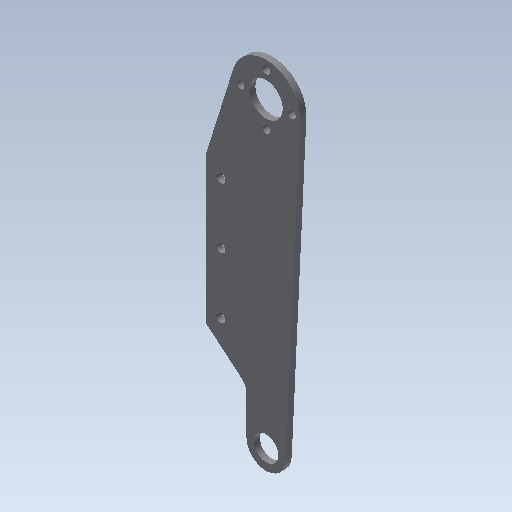
# Autodesk Inventor part: リンク_ふくらはぎ_メインフレーム_1_1
Saved by Autodesk Inventor 2020.4 (Build 244396000, 396)
## iProperties
Created: 2016-04-29
Part Number: リンク_ふくらはぎ_メインフレーム_1_1
Material: GFRP
Document SubType Name: Modeling
Designer: hiroaki
Density: 1.75 g/cm^3
Appearance: 滑らか - 淡い灰色
Mass: 9.06341 g
Surface Area: 59.5321 cm^2
Volume: 5.17909 cm^3
d0: 1.000 ul
d1: 13.000 mm
d2: 11.100 mm
d7: 3.100 mm
d8: 5.000 mm
d9: 15.000 mm
d10: 4.000 mm
d11: 40.000 mm
d12: 30.000 mm
d13: 2.000 mm
d14: 0.00 deg
d15: 2.700 mm
d16: 45.00 deg
d17: 2.700 mm
d18: 4.000 ul
d22: 1.500 mm
d23: 130.00 deg
d24: 4.000 mm
Author: hiroaki
Autodesk Inventor part; units mm, degrees
ref_plane "YZ Plane" through (0, 0, 0) normal (1, 0, 0) x (0, 1, 0)
ref_plane "XZ Plane" through (0, 0, 0) normal (0, 1, 0) x (-1, 0, 0)
ref_plane "XY Plane" through (0, 0, 0) normal (0, 0, 1) x (1, 0, 0)
derived "下半身全体像_1_1.ipt"
sketch "スケッチ1" plane through (0, 0, 0) normal (0, 0, 1) x (1, 0, 0)
  circle A0 centre (0, 0) radius 10.5 construction
  line L0 (0, 0) -> (-12, 0) construction
  arc A1 (0, 16) -> (-12, 10.583) centre (0, 0) ccw construction
  arc A2 (-12, -10.583) -> (0, -16) centre (0, 0) ccw construction
  line L1 (0, 16) -> (39.5, 16) construction
  line L2 (39.5, 16) -> (39.5, -16) construction
  line L3 (39.5, -16) -> (0, -16) construction
  circle A3 centre (1, 13.5) radius 1.35
  circle A4 centre (1, -13.5) radius 1.35 construction
  circle A5 centre (28, 13.5) radius 1.35
  circle A6 centre (28, -13.5) radius 1.35
  line L4 (1, 13.5) -> (1, -13.5) construction
  line L5 (1, -13.5) -> (28, -13.5) construction
  line L6 (1, 13.5) -> (28, 13.5) construction
  line L7 (28, 13.5) -> (28, -13.5) construction
  line L8 (0, 0) -> (1, 0) construction
  line L9 (32, 120) -> (32, 20) construction
  line L10 (0, 0) -> (0, 0) construction
  circle A7 centre (32, 120) radius 4.05
  line L11 (0, 140) -> (0, 40) construction
  circle A8 centre (0, 40) radius 4.05
  line L12 (0, 0) -> (0, -100) construction
  line L13 (32, 20) -> (32, -80) construction
  line L14 (0, 0) -> (0, 40) construction
  circle A9 centre (32, 20) radius 6.5 construction
  line L15 (32, 23.5218) -> (35.05, 21.7609) construction
  line L16 (35.05, 21.7609) -> (35.05, 18.2391) construction
  line L17 (35.05, 18.2391) -> (32, 16.4782) construction
  line L18 (32, 16.4782) -> (28.95, 18.2391) construction
  line L19 (28.95, 18.2391) -> (28.95, 21.7609) construction
  line L20 (28.95, 21.7609) -> (32, 23.5218) construction
  line L21 (21.5, 152) -> (61, 152) construction
  line L22 (61, 152) -> (61, 100.5) construction
  line L23 (61, 100.5) -> (21.5, 100.5) construction
  line L24 (21.5, 100.5) -> (21.5, 152) construction
  line L25 (21.5, 140) -> (61, 140) construction
  line L26 (16, 150.5) -> (66.5, 150.5) construction
  line L27 (66.5, 150.5) -> (66.5, 129.5) construction
  line L28 (66.5, 129.5) -> (16, 129.5) construction
  line L29 (16, 129.5) -> (16, 150.5) construction
  circle A10 centre (0, 140) radius 10.5 construction
  line L30 (-13.5, 139) -> (13.5, 139) construction
  line L31 (13.5, 139) -> (13.5, 112) construction
  line L32 (13.5, 112) -> (-13.5, 112) construction
  line L33 (-13.5, 112) -> (-13.5, 139) construction
  circle A11 centre (-13.5, 139) radius 1.35
  circle A12 centre (13.5, 139) radius 1.35
  circle A13 centre (-13.5, 112) radius 1.35
  circle A14 centre (13.5, 112) radius 1.35
  line L34 (-12, 10.583) -> (-12, -10.583) construction
  circle A15 centre (0, -100) radius 4.05
  circle A16 centre (32, -80) radius 4.05
  circle A17 centre (0, -100) radius 10.5 construction
  line L35 (32, -80) -> (0, -100) construction
  line L36 (45, -60.5) -> (77.5, -60.5) construction
  line L37 (77.5, -60.5) -> (77.5, -112) construction
  line L38 (77.5, -112) -> (45, -112) construction
  line L39 (45, -112) -> (45, -60.5) construction
  line L40 (45, -100) -> (77.5, -100) construction
  line L41 (39.5, -89.5) -> (83, -89.5) construction
  line L42 (83, -89.5) -> (83, -110.5) construction
  line L43 (83, -110.5) -> (39.5, -110.5) construction
  line L44 (39.5, -110.5) -> (39.5, -89.5) construction
  line L45 (1, -86.5) -> (28, -86.5) construction
  line L46 (28, -86.5) -> (28, -113.5) construction
  line L47 (28, -113.5) -> (1, -113.5) construction
  line L48 (1, -113.5) -> (1, -86.5) construction
  circle A18 centre (1, -86.5) radius 1.35
  circle A19 centre (1, -113.5) radius 1.35
  circle A20 centre (28, -113.5) radius 1.35
  circle A21 centre (28, -86.5) radius 1.35
  circle A22 centre (32, 20) radius 4.05
  circle A23 centre (32, 20) radius 4.05
  line L49 (10.583, 152) -> (-10.583, 152) construction
  line L50 (16, 140) -> (16, 100.5) construction
  line L51 (16, 100.5) -> (-16, 100.5) construction
  line L52 (-16, 100.5) -> (-16, 140) construction
  arc A24 (16, 140) -> (10.583, 152) centre (0, 140) ccw construction
  arc A25 (-10.583, 152) -> (-16, 140) centre (0, 140) ccw construction
  line L53 (-12, -89.417) -> (-12, -110.583) construction
  line L54 (0, -84) -> (39.5, -84) construction
  line L55 (39.5, -84) -> (39.5, -116) construction
  line L56 (39.5, -116) -> (0, -116) construction
  arc A26 (0, -84) -> (-12, -89.417) centre (0, -100) ccw construction
  arc A27 (-12, -110.583) -> (0, -116) centre (0, -100) ccw construction
  circle A28 centre (-8.5, 0) radius 1.35 construction
  circle A29 centre (0, 0) radius 8.5 construction
  line L57 (35.05, 121.7609) -> (35.05, 118.2391) construction
  line L58 (35.05, 118.2391) -> (32, 116.4782) construction
  line L59 (32, 116.4782) -> (28.95, 118.2391) construction
  line L60 (28.95, 118.2391) -> (28.95, 121.7609) construction
  line L61 (28.95, 121.7609) -> (32, 123.5218) construction
  line L62 (32, 123.5218) -> (35.05, 121.7609) construction
  circle A30 centre (0, -100) radius 6.5 construction
  circle A31 centre (0, 0) radius 5.55
  line L63 (6.4924, -100.3153) -> (11.3366, -0.5505)
  arc A32 (11.3366, -0.5505) -> (-10.8351, 3.3799) centre (0, 0) ccw
  line L64 (-10.8351, 3.3799) -> (-20, -26)
  line L65 (-20, -26) -> (-20, -74)
  arc A33 (-6.5, -100) -> (6.4924, -100.3153) centre (0, -100) ccw
  line L66 (-6.5, -100) -> (-6.5, -85.3278)
  circle A34 centre (-15, -30) radius 1.55
  line L67 (-15, -30) -> (-15, -70) construction
  circle A35 centre (-15, -70) radius 1.55
  circle A36 centre (-15, -50) radius 1.55
  line L68 (-15, -70) -> (-20, -70) construction
  line L69 (-15, -50) -> (-20, -50) construction
  line L70 (0, 152) -> (0, 140) construction
  line L71 (0, 140) -> (0, 139) construction
  circle A37 centre (-8.5, 0) radius 1.35
  line L72 (0, 0) -> (-8.5, 0) construction
  line L73 (0, 0) -> (-6.0104, 6.0104) construction
  circle A38 centre (-6.0104, 6.0104) radius 1.35
  circle A39 centre (0, -8.5) radius 1.35
  circle A40 centre (-6.0104, -6.0104) radius 1.35
  circle A41 centre (8.5, 0) radius 1.35
  circle A42 centre (6.0104, -6.0104) radius 1.35
  circle A43 centre (0, 8.5) radius 1.35
  circle A44 centre (6.0104, 6.0104) radius 1.35
  circle A45 centre (0, 0) radius 9.85 construction
  circle A46 centre (0, 0) radius 11.35 construction
  line L74 (-20, -74) -> (-6.5, -85.3278)
  line L75 (0, 0) -> (0, 8.5) construction
  point P0 (66.5, 140)
  point P1 (39.5, 0)
  point P2 (83, -100)
  point P3 (1, -100)
  point P4 (-12, -100)
  point P5 (39.5, -100)
  dimension "d1" = 13
  dimension "d2" = 11.1
  dimension "d7" = 3.1
  dimension "d8" = 5
  dimension "d9" = 15
  dimension "d10" = 4
  dimension "d11" = 40
  dimension "d12" = 30
  dimension "d15" = 2.7
  dimension "d16" = 45
  dimension "d17" = 2.7
  dimension "d20" = 360
  dimension "d22" = 1.5
  dimension "d23" = 130
  measures "d1" diameter of A30
  measures "d2" diameter of A31
  measures "d7" diameter of A34
  measures "d8" distance between parallel lines of L65 L67
  measures "d9" distance between parallel lines of L12 L67
  measures "d10" distance from line of L65.end L68
  measures "d11" distance of L67.start L67.end
  measures "d12" distance from line of A30.centre L68
  measures "d15" diameter of A37
  measures "d16" angle of L72 L73
  measures "d17" diameter of A38
  measures "d22" radial gap between concentric circles of A46 A45
  measures "d23" angle of L65 L74
extrude "押し出し1" add sketch "スケッチ1" along normal blind 2 contours A18 | A33 L66 L74 L65 L64 A32 L63 | A38 | A40 | A42 | A44
fillet "フィレット1" radius 4 1 edges at (-6.5, -85.3278, 1)
